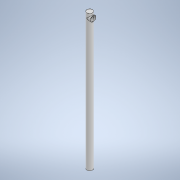
# Autodesk Inventor part: waterpip2e
Saved by Autodesk Inventor 2020 (Build 240168000, 168)
## iProperties
Created: 2019-07-25
Part Number: waterpip2e
Material: Generic
Document SubType Name: Modeling
Designer: ColinP
Density: 1 g/cm^3
Appearance: Default
Mass: 0.361255 g
Surface Area: 56.9403 cm^2
Volume: 0.361255 cm^3
Author: ColinP
Autodesk Inventor part; units mm, degrees
ref_plane "XZ Plane" through (0, 0, 0) normal (0, 1, 0) x (-1, 0, 0)
ref_plane "XY Plane" through (0, 0, 0) normal (0, 0, 1) x (1, 0, 0)
sketch "Sketch1" plane through (0, 0, 0) normal (0, 1, 0) x (-1, 0, 0)
  circle A0 centre (0, 0) radius 3.175
  circle A1 centre (0, 0) radius 3.048
  dimension "d0" = 6.35
  dimension "d1" = 6.096
  constraints: 2 centre point, 2 coincident
  measures "d0" diameter of A0
  measures "d1" diameter of A1
extrude "Extrusion1" add sketch "Sketch1" along normal blind 127
sketch "Sketch8" plane through (0, 127, 0) normal (0, 1, 0) x (1, 0, 0)
  circle A0 centre (0, 0) radius 3.175 projected
  circle A1 centre (0, 0) radius 3.048 projected
extrude "Extrusion2" add sketch "Sketch8" along normal blind 7.62
sketch "Sketch16" plane through (0, 134.62, 0) normal (0, 1, 0) x (1, 0, 0)
  circle A0 centre (0, 0) radius 3.175 projected
  circle A1 centre (0, 0) radius 3.048 projected
extrude "Extrusion3" add sketch "Sketch16" along normal blind 17.78
sketch "Sketch17" plane through (0, 152.4, 0) normal (0, 1, 0) x (1, 0, 0)
  circle A0 centre (0, 0) radius 3.175 projected
extrude "Extrusion4" add sketch "Sketch17" against normal blind 0.254
ref_plane "Work Plane2" through (12.7, 0, 0) normal (1, 0, 0) x (0, 1, 0)
sketch "Sketch18" plane through (12.7, 0, 0) normal (1, 0, 0) x (0, 1, 0)
  circle A0 centre (147.122, 0) radius 3.175
  point P0 (0, 0)
  dimension "d58" = 6.35
  constraints: 1 centre point
  measures "d58" diameter of A0
extrude "Extrusion5" cut sketch "Sketch18" against normal blind 12.7
sketch "Sketch19" plane through (0, 0, 0) normal (1, 0, 0) x (0, 0, -1)
  arc A0 (-3.175, 147.122) -> (3.175, 147.122) centre (0, 147.122) ccw projected
  circle A1 centre (0, 147.122) radius 3.175
  circle A2 centre (0, 147.122) radius 3.048
  point P0 (0, 0)
  dimension "d61" = 6.096
  constraints: 2 coincident, 1 centre point, 3 other
  measures "d61" diameter of A2
extrude "Extrusion6" add sketch "Sketch19" along normal blind 3.81
body "Solid1"
